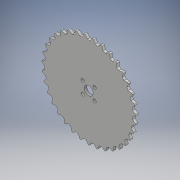
# Autodesk Inventor part: kolo 35 8,3 mm 147 dg 4,3 mm
Saved by Autodesk Inventor 2017 (Build 210142000, 142)
## iProperties
Created: 2019-08-27
Part Number: kolo 35 8,3 mm 147 dg 4,3 mm
Material: Ogólny
Document SubType Name: Modeling
Designer: patry
Density: 1 g/cm^3
Appearance: Domyślna
Author: patry
Autodesk Inventor part; units mm, degrees
ref_plane "YZ Plane" through (0, 0, 0) normal (1, 0, 0) x (0, 1, 0)
ref_plane "XZ Plane" through (0, 0, 0) normal (0, 1, 0) x (-1, 0, 0)
ref_plane "XY Plane" through (0, 0, 0) normal (0, 0, 1) x (1, 0, 0)
sketch "Szkic2" plane through (0, 0, 0) normal (0, 1, 0) x (-1, 0, 0)
  line L0 (0, 0) -> (-4.0155, -44.6163) construction
  line L1 (0, 0) -> (4.0155, -44.6163) construction
  line L2 (4.0155, -44.6163) -> (-4.0155, -44.6163) construction
  line L3 (0, 0) -> (0, -151) construction
  circle A0 centre (0, 0) radius 44.7967 construction
  line L4 (0, -48.9163) -> (2.7294, -44.7134) construction
  line L5 (0, -48.9163) -> (-2.7294, -44.7134) construction
  circle A1 centre (0, -47.159) radius 0.9571 construction
  line L6 (2.7294, -44.7134) -> (0.8027, -47.6802)
  line L7 (-2.7294, -44.7134) -> (-0.8027, -47.6802)
  arc A2 (-0.8027, -47.6802) -> (0.8027, -47.6802) centre (0, -47.159) ccw
  line L8 (-2.7294, -44.7134) -> (5.2984, -44.4822) construction
  arc A3 (2.7294, -44.7134) -> (5.2984, -44.4822) centre (0, 0) ccw
  line L9 (8.7343, -48.1302) -> (5.2984, -44.4822) construction
  line L10 (5.2984, -44.4822) -> (7.7238, -47.0573)
  arc A4 (7.7238, -47.0573) -> (9.3034, -46.7707) centre (8.4206, -46.4011) ccw
  line L11 (10.6694, -43.5075) -> (9.3034, -46.7707)
  arc A5 (10.6694, -43.5075) -> (13.1558, -42.8213) centre (0, 0) ccw
  line L12 (17.188, -45.7972) -> (13.1558, -42.8213) construction
  line L13 (13.1558, -42.8213) -> (16.0021, -44.922)
  arc A6 (16.0021, -44.922) -> (17.5052, -44.3579) centre (16.5705, -44.1519) ccw
  line L14 (18.2665, -40.9032) -> (17.5052, -44.3579)
  arc A7 (18.2665, -40.9032) -> (20.5904, -39.7841) centre (0, 0) ccw
  line L15 (25.0891, -41.9922) -> (20.5904, -39.7841) construction
  line L16 (20.5904, -39.7841) -> (23.7661, -41.3428)
  arc A8 (23.7661, -41.3428) -> (25.1443, -40.5193) centre (24.1878, -40.4836) ccw
  line L17 (25.2765, -36.9843) -> (25.1443, -40.5193)
  arc A9 (25.2765, -36.9843) -> (27.3633, -35.4682) centre (0, 0) ccw
  line L18 (32.1839, -36.8375) -> (27.3633, -35.4682) construction
  line L19 (27.3633, -35.4682) -> (30.7662, -36.4348)
  arc A10 (30.7662, -36.4348) -> (31.9752, -35.3785) centre (31.0277, -35.5141) ccw
  line L20 (31.4741, -31.8766) -> (31.9752, -35.3785)
  arc A11 (31.4741, -31.8766) -> (33.2566, -30.0123) centre (0, 0) ccw
  line L21 (38.2443, -30.4988) -> (33.2566, -30.0123) construction
  line L22 (33.2566, -30.0123) -> (36.7774, -30.3557)
  arc A12 (36.7774, -30.3557) -> (37.7784, -29.1006) centre (36.8704, -29.4031) ccw
  line L23 (36.6601, -25.7444) -> (37.7784, -29.1006)
  arc A13 (36.6601, -25.7444) -> (38.0811, -23.5918) centre (0, 0) ccw
  line L24 (43.0755, -23.1799) -> (38.0811, -23.5918) construction
  line L25 (38.0811, -23.5918) -> (41.6066, -23.301)
  arc A14 (41.6066, -23.301) -> (42.3674, -21.8873) centre (41.528, -22.3472) ccw
  line L26 (40.6678, -18.7848) -> (42.3674, -21.8873)
  arc A15 (40.6678, -18.7848) -> (41.6816, -16.413) centre (0, 0) ccw
  line L27 (46.5222, -15.116) -> (41.6816, -16.413) construction
  line L28 (41.6816, -16.413) -> (45.0986, -15.4974)
  arc A16 (45.0986, -15.4974) -> (45.5947, -13.9706) centre (44.8508, -14.5729) ccw
  line L29 (43.3684, -11.2214) -> (45.5947, -13.9706)
  arc A17 (43.3684, -11.2214) -> (43.9424, -8.7067) centre (0, 0) ccw
  line L30 (48.4736, -6.5662) -> (43.9424, -8.7067) construction
  line L31 (43.9424, -8.7067) -> (47.141, -7.1957)
  arc A18 (47.141, -7.1957) -> (47.3565, -5.6048) centre (46.7322, -6.3303) ccw
  line L32 (44.6751, -3.2973) -> (47.3565, -5.6048)
  arc A19 (44.6751, -3.2973) -> (44.7909, -0.7206) centre (0, 0) ccw
  line L33 (48.8671, 2.1946) -> (44.7909, -0.7206) construction
  line L34 (44.7909, -0.7206) -> (47.6683, 1.3373)
  arc A20 (47.6683, 1.3373) -> (47.5962, 2.9411) centre (47.1115, 2.1158) ccw
  line L35 (44.546, 4.7327) -> (47.5962, 2.9411)
  arc A21 (44.546, 4.7327) -> (44.1997, 7.2887) centre (0, 0) ccw
  line L36 (47.6899, 10.8849) -> (44.1997, 7.2887) construction
  line L37 (44.1997, 7.2887) -> (46.6634, 9.8273)
  arc A22 (46.6634, 9.8273) -> (46.3062, 11.3924) centre (45.9766, 10.4939) ccw
  line L38 (42.985, 12.6106) -> (46.3062, 11.3924)
  arc A23 (42.985, 12.6106) -> (42.188, 15.0637) centre (0, 0) ccw
  line L39 (44.9799, 19.2253) -> (42.188, 15.0637) construction
  line L40 (42.188, 15.0637) -> (44.1588, 18.0014)
  arc A24 (44.1588, 18.0014) -> (43.5278, 19.4776) centre (43.364, 18.5347) ccw
  line L41 (40.0425, 20.0832) -> (43.5278, 19.4776)
  arc A25 (40.0425, 20.0832) -> (38.8202, 22.3546) centre (0, 0) ccw
  line L42 (40.8242, 26.9479) -> (38.8202, 22.3546) construction
  line L43 (38.8202, 22.3546) -> (40.2349, 25.597)
  arc A26 (40.2349, 25.597) -> (39.3504, 26.9368) centre (39.3576, 25.9797) ccw
  line L44 (35.813, 26.9104) -> (39.3504, 26.9368)
  arc A27 (35.813, 26.9104) -> (34.2048, 28.927) centre (0, 0) ccw
  line L45 (35.3565, 33.8042) -> (34.2048, 28.927) construction
  line L46 (34.2048, 28.927) -> (35.0178, 32.3698)
  arc A28 (35.0178, 32.3698) -> (33.9083, 33.5302) centre (34.0863, 32.5898) ccw
  line L47 (30.4325, 32.8726) -> (33.9083, 33.5302)
  arc A29 (30.4325, 32.8726) -> (28.49, 34.5696) centre (0, 0) ccw
  line L48 (28.7523, 39.5741) -> (28.49, 34.5696) construction
  line L49 (28.49, 34.5696) -> (28.6752, 38.1023)
  arc A30 (28.6752, 38.1023) -> (27.3763, 39.046) centre (27.7193, 38.1524) ccw
  line L50 (24.0738, 37.7782) -> (27.3763, 39.046)
  arc A31 (24.0738, 37.7782) -> (21.8595, 39.1012) centre (0, 0) ccw
  line L51 (21.224, 44.0721) -> (21.8595, 39.1012) construction
  line L52 (21.8595, 39.1012) -> (21.4109, 42.6101)
  arc A32 (21.4109, 42.6101) -> (19.9645, 43.3067) centre (20.4615, 42.4888) ccw
  line L53 (16.9413, 41.4696) -> (19.9645, 43.3067)
  arc A33 (16.9413, 41.4696) -> (14.5264, 42.376) centre (0, 0) ccw
  line L54 (13.0135, 47.1535) -> (14.5264, 42.376) construction
  line L55 (14.5264, 42.376) -> (13.4585, 45.7484)
  arc A34 (13.4585, 45.7484) -> (11.9109, 46.1755) centre (12.546, 45.4595) ccw
  line L56 (9.2644, 43.8282) -> (11.9109, 46.1755)
  arc A35 (9.2644, 43.8282) -> (6.7265, 44.2888) centre (0, 0) ccw
  line L57 (4.3848, 48.7194) -> (6.7265, 44.2888) construction
  line L58 (6.7265, 44.2888) -> (5.0735, 47.4163)
  arc A36 (5.0735, 47.4163) -> (3.4745, 47.5603) centre (4.2273, 46.9691) ccw
  line L59 (1.2897, 44.7781) -> (3.4745, 47.5603)
  arc A37 (1.2897, 44.7781) -> (-1.2897, 44.7781) centre (0, 0) ccw
  line L60 (-4.3848, 48.7194) -> (-1.2897, 44.7781) construction
  line L61 (-1.2897, 44.7781) -> (-3.4745, 47.5603)
  arc A38 (-3.4745, 47.5603) -> (-5.0735, 47.4163) centre (-4.2273, 46.9691) ccw
  line L62 (-6.7265, 44.2888) -> (-5.0735, 47.4163)
  arc A39 (-6.7265, 44.2888) -> (-9.2644, 43.8282) centre (0, 0) ccw
  line L63 (-13.0135, 47.1535) -> (-9.2644, 43.8282) construction
  line L64 (-9.2644, 43.8282) -> (-11.9109, 46.1755)
  arc A40 (-11.9109, 46.1755) -> (-13.4585, 45.7484) centre (-12.546, 45.4595) ccw
  line L65 (-14.5264, 42.376) -> (-13.4585, 45.7484)
  arc A41 (-14.5264, 42.376) -> (-16.9413, 41.4696) centre (0, 0) ccw
  line L66 (-21.224, 44.0721) -> (-16.9413, 41.4696) construction
  line L67 (-16.9413, 41.4696) -> (-19.9645, 43.3067)
  arc A42 (-19.9645, 43.3067) -> (-21.4109, 42.6101) centre (-20.4615, 42.4888) ccw
  line L68 (-21.8595, 39.1012) -> (-21.4109, 42.6101)
  arc A43 (-21.8595, 39.1012) -> (-24.0738, 37.7782) centre (0, 0) ccw
  line L69 (-28.7523, 39.5741) -> (-24.0738, 37.7782) construction
  line L70 (-24.0738, 37.7782) -> (-27.3763, 39.046)
  arc A44 (-27.3763, 39.046) -> (-28.6752, 38.1023) centre (-27.7193, 38.1524) ccw
  line L71 (-28.49, 34.5696) -> (-28.6752, 38.1023)
  arc A45 (-28.49, 34.5696) -> (-30.4325, 32.8726) centre (0, 0) ccw
  line L72 (-35.3565, 33.8042) -> (-30.4325, 32.8726) construction
  line L73 (-30.4325, 32.8726) -> (-33.9083, 33.5302)
  arc A46 (-33.9083, 33.5302) -> (-35.0178, 32.3698) centre (-34.0863, 32.5898) ccw
  line L74 (-34.2048, 28.927) -> (-35.0178, 32.3698)
  arc A47 (-34.2048, 28.927) -> (-35.813, 26.9104) centre (0, 0) ccw
  line L75 (-40.8242, 26.9479) -> (-35.813, 26.9104) construction
  line L76 (-35.813, 26.9104) -> (-39.3504, 26.9368)
  arc A48 (-39.3504, 26.9368) -> (-40.2349, 25.597) centre (-39.3576, 25.9797) ccw
  line L77 (-38.8202, 22.3546) -> (-40.2349, 25.597)
  arc A49 (-38.8202, 22.3546) -> (-40.0425, 20.0832) centre (0, 0) ccw
  line L78 (-44.9799, 19.2253) -> (-40.0425, 20.0832) construction
  line L79 (-40.0425, 20.0832) -> (-43.5278, 19.4776)
  arc A50 (-43.5278, 19.4776) -> (-44.1588, 18.0014) centre (-43.364, 18.5347) ccw
  line L80 (-42.188, 15.0637) -> (-44.1588, 18.0014)
  arc A51 (-42.188, 15.0637) -> (-42.985, 12.6106) centre (0, 0) ccw
  line L81 (-47.6899, 10.8849) -> (-42.985, 12.6106) construction
  line L82 (-42.985, 12.6106) -> (-46.3062, 11.3924)
  arc A52 (-46.3062, 11.3924) -> (-46.6634, 9.8273) centre (-45.9766, 10.4939) ccw
  line L83 (-44.1997, 7.2887) -> (-46.6634, 9.8273)
  arc A53 (-44.1997, 7.2887) -> (-44.546, 4.7327) centre (0, 0) ccw
  line L84 (-48.8671, 2.1946) -> (-44.546, 4.7327) construction
  line L85 (-44.546, 4.7327) -> (-47.5962, 2.9411)
  arc A54 (-47.5962, 2.9411) -> (-47.6683, 1.3373) centre (-47.1115, 2.1158) ccw
  line L86 (-44.7909, -0.7206) -> (-47.6683, 1.3373)
  arc A55 (-44.7909, -0.7206) -> (-44.6751, -3.2973) centre (0, 0) ccw
  line L87 (-48.4736, -6.5662) -> (-44.6751, -3.2973) construction
  line L88 (-44.6751, -3.2973) -> (-47.3565, -5.6048)
  arc A56 (-47.3565, -5.6048) -> (-47.141, -7.1957) centre (-46.7322, -6.3303) ccw
  line L89 (-43.9424, -8.7067) -> (-47.141, -7.1957)
  arc A57 (-43.9424, -8.7067) -> (-43.3684, -11.2214) centre (0, 0) ccw
  line L90 (-46.5222, -15.116) -> (-43.3684, -11.2214) construction
  line L91 (-43.3684, -11.2214) -> (-45.5947, -13.9706)
  arc A58 (-45.5947, -13.9706) -> (-45.0986, -15.4974) centre (-44.8508, -14.5729) ccw
  line L92 (-41.6816, -16.413) -> (-45.0986, -15.4974)
  arc A59 (-41.6816, -16.413) -> (-40.6678, -18.7848) centre (0, 0) ccw
  line L93 (-43.0755, -23.1799) -> (-40.6678, -18.7848) construction
  line L94 (-40.6678, -18.7848) -> (-42.3674, -21.8873)
  arc A60 (-42.3674, -21.8873) -> (-41.6066, -23.301) centre (-41.528, -22.3472) ccw
  line L95 (-38.0811, -23.5918) -> (-41.6066, -23.301)
  arc A61 (-38.0811, -23.5918) -> (-36.6601, -25.7444) centre (0, 0) ccw
  line L96 (-38.2443, -30.4988) -> (-36.6601, -25.7444) construction
  line L97 (-36.6601, -25.7444) -> (-37.7784, -29.1006)
  arc A62 (-37.7784, -29.1006) -> (-36.7774, -30.3557) centre (-36.8704, -29.4031) ccw
  line L98 (-33.2566, -30.0123) -> (-36.7774, -30.3557)
  arc A63 (-33.2566, -30.0123) -> (-31.4741, -31.8766) centre (0, 0) ccw
  line L99 (-32.1839, -36.8375) -> (-31.4741, -31.8766) construction
  line L100 (-31.4741, -31.8766) -> (-31.9752, -35.3785)
  arc A64 (-31.9752, -35.3785) -> (-30.7662, -36.4348) centre (-31.0277, -35.5141) ccw
  line L101 (-27.3633, -35.4682) -> (-30.7662, -36.4348)
  arc A65 (-27.3633, -35.4682) -> (-25.2765, -36.9843) centre (0, 0) ccw
  line L102 (-25.0891, -41.9922) -> (-25.2765, -36.9843) construction
  line L103 (-25.2765, -36.9843) -> (-25.1443, -40.5193)
  arc A66 (-25.1443, -40.5193) -> (-23.7661, -41.3428) centre (-24.1878, -40.4836) ccw
  line L104 (-20.5904, -39.7841) -> (-23.7661, -41.3428)
  arc A67 (-20.5904, -39.7841) -> (-18.2665, -40.9032) centre (0, 0) ccw
  line L105 (-17.188, -45.7972) -> (-18.2665, -40.9032) construction
  line L106 (-18.2665, -40.9032) -> (-17.5052, -44.3579)
  arc A68 (-17.5052, -44.3579) -> (-16.0021, -44.922) centre (-16.5705, -44.1519) ccw
  line L107 (-13.1558, -42.8213) -> (-16.0021, -44.922)
  arc A69 (-13.1558, -42.8213) -> (-10.6694, -43.5075) centre (0, 0) ccw
  line L108 (-8.7343, -48.1302) -> (-10.6694, -43.5075) construction
  line L109 (-10.6694, -43.5075) -> (-9.3034, -46.7707)
  arc A70 (-9.3034, -46.7707) -> (-7.7238, -47.0573) centre (-8.4206, -46.4011) ccw
  line L110 (-5.2984, -44.4822) -> (-7.7238, -47.0573)
  arc A71 (-5.2984, -44.4822) -> (-2.7294, -44.7134) centre (0, 0) ccw
  dimension "d19" = 8.0311
  dimension "d20" = 4.0155
  dimension "d21" = 10.286
  dimension "d22" = 4.3
  dimension "d23" = 147
  dimension "d24" = 147
  dimension "d26" = 8.0311
  dimension "d44" = 1.7573
  constraints: 222 end point, 146 point on circle, 72 centre point, 38 point on line, 2 coincident, 2 tangent, 1 concentric, 1 equal length, 1 vertical, 2 other
  measures "d19" distance of L1.end L0.end
  measures "d20" distance from line of L1.end L3
  measures "d21" angle of L1 L0
  measures "d22" distance from line of L2 L4.start
  measures "d23" angle of L3 L4
  measures "d24" angle of L3 L5
  measures "d26" distance of L8.end L5.end
  measures "d44" distance of L4.start point (0, -47.159)
sketch "Szkic3" plane through (0, 0, 0) normal (0, 1, 0) x (-1, 0, 0)
  circle A0 centre (0, 0) radius 8.5 construction
  line L0 (-6.0104, 6.0104) -> (6.0104, 6.0104) construction
  line L1 (6.0104, 6.0104) -> (6.0104, -6.0104) construction
  line L2 (6.0104, -6.0104) -> (-6.0104, -6.0104) construction
  line L3 (-6.0104, -6.0104) -> (-6.0104, 6.0104) construction
  line L4 (-6.0104, 6.0104) -> (6.0104, -6.0104) construction
  line L5 (6.0104, 6.0104) -> (-6.0104, -6.0104) construction
  dimension "d37" = 17
  constraints: 12 end point, 5 coincident, 2 midpoint, 2 parallel, 2 perpendicular, 1 horizontal, 3 other
extrude "Wyciągnięcie proste2" add sketch "Szkic2" along normal blind 2.5
hole "Otwór1" at (-6.0104, 0, -6.0104) at (6.0104, 0, -6.0104) at (6.0104, 0, 6.0104) at (-6.0104, 0, 6.0104) direction (0, 1, 0) diameter 3.3 end through all
sketch "Szkic4" plane through (0, 0, 0) normal (0, -1, 0) x (1, 0, 0)
  point P0 (0, 0)
  point P1 (0, 0)
  constraints: 1 coincident
hole "Otwór2" at (0, 0, 0) direction (0, 1, 0) diameter 9 end through all
equation "\"d19\" = dl_przeskoku"
equation "\"d20\" = 0.5 * d19"
equation "\"d23\" = kat_zeba"
equation "\"d24\" = kat_zeba"
equation "\"d26\" = dl_przeskoku"
equation "\"kat\" = 360deg"
equation "\"kat_zeba\" = 147deg"
equation "\"wys_zeba\" = 5"
equation "\"odl_osi_zeba\" = 2.366"
equation "\"dl_ogniwa\" = 8.3"
equation "\"dl_przeskoku\" = 8.031082"
